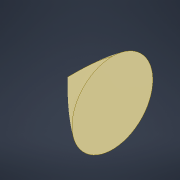
# Autodesk Inventor part: sincos half
Saved by Autodesk Inventor 2022 (Build 260153000, 153)
## iProperties
Created: 2021-06-07
Part Number: sincos half
Material: Generic
Document SubType Name: Modeling
Designer: sidsa
Density: 1 g/cm^3
Appearance: Gold - Metal
Author: sidsa
## iProperties of the stored document sincos half_3DPrint.ipt
Created: 2021-06-07
Part Number: sincos half_3DPrint
Material: Generic
Document SubType Name: Modeling
Designer: sidsa
Density: 1 g/cm^3
Appearance: Default
Author: sidsa
Autodesk Inventor part; units mm, degrees
ref_plane "YZ Plane" through (0, 0, 0) normal (1, 0, 0) x (0, 1, 0)
ref_plane "XZ Plane" through (0, 0, 0) normal (0, 1, 0) x (-1, 0, 0)
ref_plane "XY Plane" through (0, 0, 0) normal (0, 0, 1) x (1, 0, 0)
sketch "Sketch1" plane through (0, 0, 0) normal (0, 0, 1) x (1, 0, 0)
  spline S0 degree 5 poles (0, 0) (4.952, 4.9427) (9.6801, 9.7091) (14.9997, 14.5834) (24.6572, 22.3082) (37.0549, 26.2035) (42.7392, 26.2035) (55.1369, 22.3082) (64.7944, 14.5834) (70.114, 9.7091) (74.8421, 4.9427) (79.7941, 0) knots 0 0 0 0 0 0 0.35722 0.35722 0.35722 0.64278 0.64278 0.64278 1 1 1 1 1 1
  spline S1 degree 5 poles (0, 25.4) (10.0476, 25.3951) (18.5836, 20.4694) (26.5285, 13.3041) (32.8905, 7.0175) (39.8982, -0.0012) knots 0 0 0 0 0 0 1 1 1 1 1 1
  line L0 (0, 0) -> (39.8982, 0)
  line L1 (19.9487, 17.9606) -> (19.9491, 0)
  point P0 (19.9487, 17.9606)
  constraints: 4 end point, 1 horizontal, 1 midpoint, 8 other
revolve "Revolution2" add sketch "Sketch1" angle 360 about axis through (0, 0, 0) along (1, 0, 0) contours S0 L1 L0
equation "curve S0 of \"Sketch1\": x = t; y = 1 in * sin(t * 180 / 3.1415); t from d0 to d1"
equation "curve S1 of \"Sketch1\": x = t; y = cos(t * 180 / 3.1415); t from d2 to d3"
body "Solid2"
